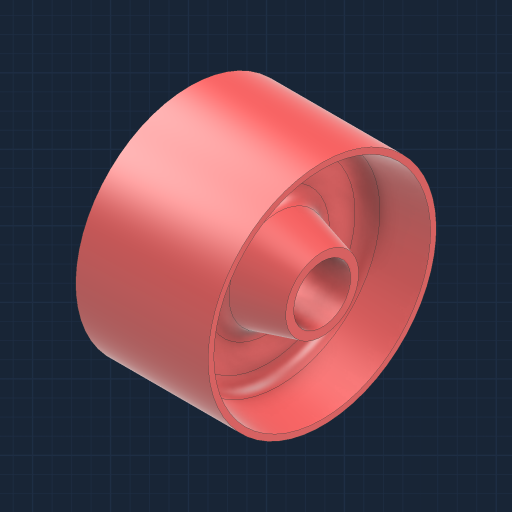
# Autodesk Inventor part: 04-roller
Saved by Autodesk Inventor 2024 (Build 280153000, 153)
## iProperties
Created: 2025-03-09
Part Number: 04-roller
Material: Stainless Steel
Document SubType Name: Modeling
Designer: DuctopwH
Density: 8 g/cm^3
Appearance: Semi-Polished
Author: DuctopwH
Autodesk Inventor part; units mm, degrees
ref_plane "YZ Plane" through (0, 0, 0) normal (1, 0, 0) x (0, 1, 0)
ref_plane "XZ Plane" through (0, 0, 0) normal (0, 1, 0) x (-1, 0, 0)
ref_plane "XY Plane" through (0, 0, 0) normal (0, 0, 1) x (1, 0, 0)
sketch "Sketch1" plane through (0, 0, 0) normal (0, 0, 1) x (1, 0, 0)
  line L0 (-26.0293, 0) -> (0, 0)
  line L1 (0, 0) -> (26.0293, 0)
  line L2 (0, 0) -> (0, 50) construction
  line L3 (0, 50) -> (29, 50)
  line L4 (29, 50) -> (29, 47.5)
  line L5 (29, 47.5) -> (5, 43.5)
  line L6 (5, 43.5) -> (5, 22.5)
  line L7 (5, 22.5) -> (29, 16)
  line L8 (29, 16) -> (29, 12.5)
  line L9 (29, 12.5) -> (0, 12.5)
  line L10 (0, 50) -> (-29, 50)
  line L11 (-29, 47.5) -> (-5, 43.5)
  line L12 (-5, 43.5) -> (-5, 22.5)
  line L13 (-5, 22.5) -> (-29, 16)
  line L14 (-29, 16) -> (-29, 12.5)
  line L15 (-29, 12.5) -> (0, 12.5)
  line L16 (-29, 50) -> (-29, 47.5)
  point P0 (14.5, 12.5)
  point P1 (-14.5, 12.5)
  point P2 (-5, 33)
  dimension "d0" = 100
  dimension "d1" = 95
  dimension "d2" = 87
  dimension "d3" = 45
  dimension "d4" = 25
  dimension "d5" = 32
  dimension "d6" = 58
  dimension "d7" = 10
  constraints: 34 end point, 7 symmetric about line, 4 collinear, 2 horizontal, 2 midpoint, 2 perpendicular, 1 parallel, 1 point on line, 1 vertical
  measures "d0" diameter of L3 L1
  measures "d1" diameter of L4.end L1
  measures "d2" diameter of L5.end L1
  measures "d3" diameter of L6.end L1
  measures "d4" diameter of point (14.5, 12.5) L1
  measures "d5" diameter of L7.end L1
  measures "d6" distance of L3.end L10.end
  measures "d7" distance from line of point (-5, 33) L6
revolve "Revolution1" add sketch "Sketch1" angle 360 about axis through (-26.0293, 0, 0) along (1, 0, 0)
fillet "Fillet1" radius 6 4 edges at (5, -43.5, 0) (5, -22.5, 0) (-5, -43.5, 0) (-5, -22.5, 0)
body "Solid1"
